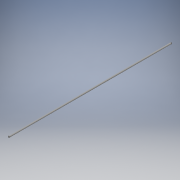
# Autodesk Inventor part: 8M 900mm threaded rod
Saved by Autodesk Inventor 2018 (Build 220112000, 112)
## iProperties
Created: 2017-11-24
Part Number: 8M 900mm threaded rod
Material: Generic
Document SubType Name: Modeling
Designer: g
Density: 1 g/cm^3
Appearance: Default
Author: g
Autodesk Inventor part; units mm, degrees
ref_plane "YZ Plane" through (0, 0, 0) normal (1, 0, 0) x (0, 1, 0)
ref_plane "XZ Plane" through (0, 0, 0) normal (0, 1, 0) x (-1, 0, 0)
ref_plane "XY Plane" through (0, 0, 0) normal (0, 0, 1) x (1, 0, 0)
sketch "Sketch1" plane through (0, 0, 0) normal (0, 1, 0) x (-1, 0, 0)
  circle A0 centre (0, 0) radius 4
  dimension "d0" = 8
  constraints: 1 centre point, 1 coincident
  measures "d0" diameter of A0
extrude "Extrusion1" add sketch "Sketch1" along normal blind 900
thread "Thread1" size "M8x1" class "6g" standard "ISO Metric profile" full length
sketch "Sketch2" plane through (0, 900, 0) normal (0, 1, 0) x (1, 0, 0)
  arc A0 (-2, -1.5) -> (-2, 1.5) centre (0, 0) ccw
  line L0 (-2, -1.5) -> (-2, 1.5)
  dimension "d5" = 5
  dimension "d6" = 2
  constraints: 2 end point, 2 point on circle, 1 centre point, 1 coincident, 1 vertical
  measures "d5" diameter of A0
  measures "d6" distance from line of point (0, 0) L0
extrude "Extrusion2" cut sketch "Sketch2" against normal blind 5
body "Solid1"
